Autodesk Inventor part; units mm, degrees
(part 2 of 2)
  measures "d144" distance between parallel lines of L36 L56
  measures "d146" radius of A87
  measures "d147" diameter of A91
  measures "d148" distance between parallel lines of L36 L60
  measures "d149" distance between parallel lines of L22 L61
  measures "d150" distance between parallel lines of L31 L62
  measures "d151" radius of A94
  measures "d153" distance between parallel lines of L21 L63
  measures "d154" distance between parallel lines of L22 L64
  measures "d155" distance between parallel lines of L38 L65
  measures "d156" distance between parallel lines of L23 L66
  measures "d157" radius of A101
  measures "d158" radius of A107
  measures "d159" diameter of A108
  measures "d160" distance between parallel lines of L32 L68
  measures "d161" distance between parallel lines of L28 L69
  measures "d162" distance between parallel lines of L29 L70
  measures "d163" distance between parallel lines of L30 L71
  measures "d164" radius of A112
  measures "d170" distance between parallel lines of L26 L73
  measures "d171" distance between parallel lines of L29 L74
  measures "d172" radius of A117
  measures "d173" radius of A120
  measures "d174" diameter of A122
  measures "d175" distance between parallel lines of L23 L76
  measures "d176" distance between parallel lines of L27 L77
  measures "d177" distance between parallel lines of L26 L78
  measures "d178" distance between parallel lines of L25 L79
extrude "Extrusion3" cut sketch "Sketch2" against normal blind 4.7625
sketch "Sketch4" plane through (0, 4.7625, 0) normal (0, 1, 0) x (1, 0, 0)
  arc A0 (-39.1165, 26.3357) -> (-36.1072, 19.7253) centre (-34.8076, 24.3071) ccw projected
  line L0 (-39.1165, 26.3357) -> (-33.046, 39.2298) projected
  arc A1 (-24.1207, 38.3715) -> (-33.046, 39.2298) centre (-28.7371, 37.2012) ccw projected
  line L1 (-24.1207, 38.3715) -> (-20.9678, 25.9338) projected
  arc A2 (-25.5116, 20.0016) -> (-20.9678, 25.9338) centre (-25.5843, 24.7636) ccw projected
  arc A3 (-25.5116, 20.0016) -> (-29.2434, 18.9092) centre (-25.4, 12.7) ccw projected
  arc A4 (-34.2566, 18.9092) -> (-29.2434, 18.9092) centre (-31.75, 22.9587) ccw projected
  arc A5 (-34.2566, 18.9092) -> (-36.1072, 19.7253) centre (-38.1, 12.7) ccw projected
  arc A6 (10.7493, 83.4364) -> (18.6675, 82.9982) centre (14.8541, 85.8512) ccw projected
  line L2 (10.7493, 83.4364) -> (3.5125, 95.7378) projected
  arc A7 (5.2361, 102.2771) -> (3.5125, 95.7378) centre (7.6174, 98.1526) ccw projected
  line L3 (5.2361, 102.2771) -> (9.4199, 104.6926) projected
  arc A8 (13.3535, 105.0706) -> (9.4199, 104.6926) centre (11.8012, 100.5682) ccw projected
  arc A9 (13.3535, 105.0706) -> (19.7173, 105.0706) centre (16.5354, 114.3) ccw projected
  arc A10 (23.6509, 104.6926) -> (19.7173, 105.0706) centre (21.2696, 100.5682) ccw projected
  line L4 (23.6509, 104.6926) -> (26.8599, 102.8399) projected
  arc A11 (28.292, 95.8625) -> (26.8599, 102.8399) centre (24.4786, 98.7155) ccw projected
  line L5 (28.292, 95.8625) -> (18.6675, 82.9982) projected
  arc A12 (33.2042, 118.4244) -> (33.2042, 110.1756) centre (35.5854, 114.3) ccw projected
  line L6 (33.2042, 118.4244) -> (34.5005, 119.1729) projected
  arc A13 (37.5333, 119.7662) -> (34.5005, 119.1729) centre (36.8818, 115.0485) ccw projected
  arc A14 (37.5333, 119.7662) -> (40.1924, 119.8887) centre (38.5324, 127) ccw projected
  arc A15 (46.0375, 115.2508) -> (40.1924, 119.8887) centre (41.275, 115.2508) ccw projected
  line L7 (46.0375, 115.2508) -> (46.0375, 114.3) projected
  arc A16 (39.6449, 108.8173) -> (46.0375, 114.3) centre (40.49, 114.3) ccw projected
  arc A17 (39.6449, 108.8173) -> (37.5333, 108.8338) centre (38.5324, 101.6) ccw projected
  arc A18 (34.5005, 109.4271) -> (37.5333, 108.8338) centre (36.8818, 113.5515) ccw projected
  line L8 (34.5005, 109.4271) -> (33.2042, 110.1756) projected
  arc A19 (-0.6991, 113.9403) -> (2.8442, 111.8946) centre (1.6631, 113.9403) ccw projected
  line L9 (-0.6991, 113.9403) -> (-0.6991, 114.6597) projected
  arc A20 (2.8442, 116.7054) -> (-0.6991, 114.6597) centre (1.6631, 114.6597) ccw projected
  line L10 (2.8442, 116.7054) -> (3.4671, 116.3457) projected
  arc A21 (3.4671, 112.2543) -> (3.4671, 116.3457) centre (2.286, 114.3) ccw projected
  line L11 (3.4671, 112.2543) -> (2.8442, 111.8946) projected
  line L12 (41.275, 207.9625) -> (30.1653, 207.9625) projected
  arc A22 (26.0308, 215.0888) -> (30.1653, 207.9625) centre (30.1653, 212.725) ccw projected
  line L13 (26.0308, 215.0888) -> (37.1405, 234.5209) projected
  arc A23 (46.0375, 232.1571) -> (37.1405, 234.5209) centre (41.275, 232.1571) ccw projected
  line L14 (46.0375, 232.1571) -> (46.0375, 212.725) projected
  arc A24 (41.275, 207.9625) -> (46.0375, 212.725) centre (41.275, 212.725) ccw projected
  line L15 (-18.8398, 318.7446) -> (-15.9012, 313.5602) projected
  arc A25 (-18.9742, 306.5711) -> (-15.9012, 313.5602) centre (-20.0445, 311.2118) ccw projected
  line L16 (-18.9742, 306.5711) -> (-23.6444, 305.494) projected
  arc A26 (-29.3048, 311.4041) -> (-23.6444, 305.494) centre (-24.7146, 310.1347) ccw projected
  line L17 (-29.3048, 311.4041) -> (-27.5732, 317.6656) projected
  arc A27 (-18.8398, 318.7446) -> (-27.5732, 317.6656) centre (-22.983, 316.3962) ccw projected
  arc A28 (-53.975, 336.3341) -> (-58.7375, 331.5716) centre (-53.975, 331.5716) ccw projected
  line L18 (-53.975, 336.3341) -> (-47.8591, 336.3341) projected
  arc A29 (-43.4942, 333.4766) -> (-47.8591, 336.3341) centre (-47.8591, 331.5716) ccw projected
  arc A30 (-43.4942, 333.4766) -> (-38.0327, 326.2997) centre (-26.0346, 341.0966) ccw projected
  arc A31 (-36.442, 321.3311) -> (-38.0327, 326.2997) centre (-41.0322, 322.6005) ccw projected
  line L19 (-36.442, 321.3311) -> (-40.7412, 305.7855) projected
  arc A32 (-43.8878, 302.5165) -> (-40.7412, 305.7855) centre (-45.3314, 307.055) ccw projected
  line L20 (-43.8878, 302.5165) -> (-52.3056, 299.8389) projected
  arc A33 (-52.3056, 299.8389) -> (-52.4379, 299.7953) centre (-50.2604, 293.4095) ccw projected
  arc A34 (-58.7375, 304.3029) -> (-52.4379, 299.7953) centre (-53.975, 304.3029) ccw projected
  line L21 (-58.7375, 304.3029) -> (-58.7375, 331.5716) projected
  arc A35 (5.8207, 343.1819) -> (9.0856, 344.1221) centre (6.222, 347.9275) ccw projected
  line L22 (5.8207, 343.1819) -> (-3.8863, 344.0029) projected
  arc A36 (-7.9949, 347.2181) -> (-3.8863, 344.0029) centre (-3.485, 348.7485) ccw projected
  arc A37 (-7.9949, 347.2181) -> (-14.358, 356.1485) centre (-26.0346, 341.0966) ccw projected
  arc A38 (-16.0554, 361.0817) -> (-14.358, 356.1485) centre (-11.4389, 359.9115) ccw projected
  line L23 (-16.0554, 361.0817) -> (-13.3658, 371.6918) projected
  arc A39 (-4.8645, 373.2765) -> (-13.3658, 371.6918) centre (-8.7493, 370.5216) ccw projected
  line L24 (-4.8645, 373.2765) -> (10.8092, 351.1749) projected
  arc A40 (9.5261, 344.431) -> (10.8092, 351.1749) centre (6.9244, 348.42) ccw projected
  arc A41 (9.5261, 344.431) -> (9.0856, 344.1221) centre (13.904, 337.7188) ccw projected
  arc A42 (-9.4515, 321.4974) -> (-1.2033, 321.431) centre (-5.3082, 323.8458) ccw projected
  line L25 (-9.4515, 321.4974) -> (-11.1297, 324.4583) projected
  arc A43 (-10.796, 329.6646) -> (-11.1297, 324.4583) centre (-6.9864, 326.8067) ccw projected
  arc A44 (-10.796, 329.6646) -> (-9.2793, 332.0323) centre (-26.0346, 341.0966) ccw projected
  arc A45 (-4.6891, 334.5118) -> (-9.2793, 332.0323) centre (-5.0904, 329.7662) ccw projected
  line L26 (-4.6891, 334.5118) -> (-1.5787, 334.2487) projected
  arc A46 (2.1248, 327.0883) -> (-1.5787, 334.2487) centre (-1.9801, 329.5032) ccw projected
  line L27 (2.1248, 327.0883) -> (-1.2033, 321.431) projected
  arc A47 (19.7173, 301.3294) -> (13.3535, 301.3294) centre (16.5354, 292.1) ccw projected
  arc A48 (9.4199, 301.7074) -> (13.3535, 301.3294) centre (11.8012, 305.8318) ccw projected
  line L28 (9.4199, 301.7074) -> (5.2361, 304.1229) projected
  arc A49 (3.5125, 310.6622) -> (5.2361, 304.1229) centre (7.6174, 308.2474) ccw projected
  line L29 (3.5125, 310.6622) -> (10.7493, 322.9636) projected
  arc A50 (18.6675, 323.4018) -> (10.7493, 322.9636) centre (14.8541, 320.5488) ccw projected
  line L30 (18.6675, 323.4018) -> (28.292, 310.5375) projected
  arc A51 (26.8599, 303.5601) -> (28.292, 310.5375) centre (24.4786, 307.6845) ccw projected
  line L31 (26.8599, 303.5601) -> (23.6509, 301.7074) projected
  arc A52 (19.7173, 301.3294) -> (23.6509, 301.7074) centre (21.2696, 305.8318) ccw projected
  arc A53 (9.6134, 220.0272) -> (17.8824, 220.0272) centre (13.7479, 222.3909) ccw projected
  line L32 (9.6134, 220.0272) -> (4.0277, 229.7971) projected
  arc A54 (4.342, 235.0047) -> (4.0277, 229.7971) centre (8.1622, 232.1609) ccw projected
  arc A55 (4.342, 235.0047) -> (7.636, 242.1522) centre (-10.9389, 246.38) ccw projected
  arc A56 (11.391, 245.774) -> (7.636, 242.1522) centre (12.2798, 241.0952) ccw projected
  line L33 (11.391, 245.774) -> (25.0344, 248.3657) projected
  arc A57 (30.0577, 241.3231) -> (25.0344, 248.3657) centre (25.9232, 243.6869) ccw projected
  line L34 (30.0577, 241.3231) -> (17.8824, 220.0272) projected
  arc A58 (30.1653, 198.4375) -> (26.0308, 191.3112) centre (30.1653, 193.675) ccw projected
  line L35 (30.1653, 198.4375) -> (41.275, 198.4375) projected
  arc A59 (46.0375, 193.675) -> (41.275, 198.4375) centre (41.275, 193.675) ccw projected
  line L36 (46.0375, 193.675) -> (46.0375, 174.2429) projected
  arc A60 (37.1405, 171.8791) -> (46.0375, 174.2429) centre (41.275, 174.2429) ccw projected
  line L37 (37.1405, 171.8791) -> (26.0308, 191.3112) projected
  arc A61 (-58.7375, 140.2762) -> (-54.2943, 135.5245) centre (-53.975, 140.2762) ccw projected
  line L38 (-58.7375, 140.2762) -> (-58.7375, 193.675) projected
  arc A62 (-53.975, 198.4375) -> (-58.7375, 193.675) centre (-53.975, 193.675) ccw projected
  line L39 (-53.975, 198.4375) -> (-52.8865, 198.4375) projected
  arc A63 (-49.7125, 197.2256) -> (-52.8865, 198.4375) centre (-52.8865, 193.675) ccw projected
  arc A64 (-49.7125, 197.2256) -> (-45.8257, 195.3193) centre (-44.3715, 203.2) ccw projected
  arc A65 (-42.9243, 193.5516) -> (-45.8257, 195.3193) centre (-46.69, 190.6359) ccw projected
  line L40 (-42.9243, 193.5516) -> (-28.0657, 174.361) projected
  arc A66 (-27.6529, 169.1603) -> (-28.0657, 174.361) centre (-31.8314, 171.4453) ccw projected
  arc A67 (-27.6529, 169.1603) -> (-29.5057, 155.7567) centre (-10.9389, 160.02) ccw projected
  arc A68 (-31.3139, 150.863) -> (-29.5057, 155.7567) centre (-34.1474, 154.6908) ccw projected
  line L41 (-31.3139, 150.863) -> (-50.8212, 136.4228) projected
  arc A69 (-54.0935, 135.5084) -> (-50.8212, 136.4228) centre (-53.6548, 140.2507) ccw projected
  arc A70 (-54.0935, 135.5084) -> (-54.2943, 135.5245) centre (-54.8316, 127.5288) ccw projected
  arc A71 (-11.1297, 81.9417) -> (-10.796, 76.7354) centre (-6.9864, 79.5933) ccw projected
  line L42 (-11.1297, 81.9417) -> (-9.4515, 84.9026) projected
  arc A72 (-1.2033, 84.969) -> (-9.4515, 84.9026) centre (-5.3082, 82.5542) ccw projected
  line L43 (-1.2033, 84.969) -> (2.1248, 79.3117) projected
  arc A73 (-1.5787, 72.1513) -> (2.1248, 79.3117) centre (-1.9801, 76.8968) ccw projected
  line L44 (-1.5787, 72.1513) -> (-4.6891, 71.8882) projected
  arc A74 (-9.2793, 74.3677) -> (-4.6891, 71.8882) centre (-5.0904, 76.6338) ccw projected
  arc A75 (-9.2793, 74.3677) -> (-10.796, 76.7354) centre (-26.0346, 65.3034) ccw projected
  arc A76 (-53.975, 60.5409) -> (-58.7375, 55.7784) centre (-53.975, 55.7784) ccw projected
  line L45 (-53.975, 60.5409) -> (-47.8591, 60.5409) projected
  arc A77 (-43.4942, 57.6834) -> (-47.8591, 60.5409) centre (-47.8591, 55.7784) ccw projected
  arc A78 (-43.4942, 57.6834) -> (-40.3657, 52.7526) centre (-26.0346, 65.3034) ccw projected
  arc A79 (-39.6396, 47.5863) -> (-40.3657, 52.7526) centre (-43.9484, 49.6149) ccw projected
  line L46 (-39.6396, 47.5863) -> (-49.6661, 26.2893) projected
  arc A80 (-58.7375, 28.3179) -> (-49.6661, 26.2893) centre (-53.975, 28.3179) ccw projected
  line L47 (-58.7375, 28.3179) -> (-58.7375, 55.7784) projected
  arc A81 (-13.3658, 34.7082) -> (-4.8645, 33.1235) centre (-8.7493, 35.8784) ccw projected
  line L48 (-13.3658, 34.7082) -> (-16.0554, 45.3183) projected
  arc A82 (-14.358, 50.2515) -> (-16.0554, 45.3183) centre (-11.4389, 46.4885) ccw projected
  arc A83 (-14.358, 50.2515) -> (-7.9949, 59.1819) centre (-26.0346, 65.3034) ccw projected
  arc A84 (-3.8863, 62.3971) -> (-7.9949, 59.1819) centre (-3.485, 57.6515) ccw projected
  line L49 (-3.8863, 62.3971) -> (5.8207, 63.2181) projected
  arc A85 (9.0856, 62.2779) -> (5.8207, 63.2181) centre (6.222, 58.4725) ccw projected
  arc A86 (9.0856, 62.2779) -> (9.5261, 61.969) centre (13.904, 68.6812) ccw projected
  arc A87 (10.8092, 55.2251) -> (9.5261, 61.969) centre (6.9244, 57.98) ccw projected
  line L50 (10.8092, 55.2251) -> (-4.8645, 33.1235) projected
  arc A88 (-12.0658, 137.7103) -> (-15.5991, 141.5488) centre (-16.7641, 136.931) ccw projected
  line L51 (-12.0658, 137.7103) -> (-11.3718, 133.5261) projected
  arc A89 (-11.8825, 130.4783) -> (-11.3718, 133.5261) centre (-16.0701, 132.7468) ccw projected
  arc A90 (-11.8825, 130.4783) -> (-11.2268, 122.5178) centre (-5.4616, 127) ccw projected
  arc A91 (-10.2241, 119.5947) -> (-11.2268, 122.5178) centre (-14.9866, 119.5947) ccw projected
  line L52 (-10.2241, 119.5947) -> (-10.2241, 113.5718) projected
  arc A92 (-16.0569, 108.9311) -> (-10.2241, 113.5718) centre (-14.9866, 113.5718) ccw projected
  line L53 (-16.0569, 108.9311) -> (-30.7922, 112.3296) projected
  arc A93 (-33.2127, 113.7305) -> (-30.7922, 112.3296) centre (-29.7219, 116.9703) ccw projected
  arc A94 (-33.2127, 113.7305) -> (-36.1128, 115.5703) centre (-38.1579, 109.1408) ccw projected
  line L54 (-36.1128, 115.5703) -> (-44.4253, 118.2144) projected
  arc A95 (-47.3989, 124.5331) -> (-44.4253, 118.2144) centre (-42.9817, 122.7528) ccw projected
  arc A96 (-47.3989, 124.5331) -> (-46.9843, 125.9045) centre (-54.8316, 127.5288) ccw projected
  arc A97 (-45.1542, 128.7671) -> (-46.9843, 125.9045) centre (-42.3206, 124.9392) ccw projected
  line L55 (-45.1542, 128.7671) -> (-25.6468, 143.2073) projected
  arc A98 (-20.4384, 143.5075) -> (-25.6468, 143.2073) centre (-22.8133, 139.3794) ccw projected
  arc A99 (-20.4384, 143.5075) -> (-15.5991, 141.5488) centre (-10.9389, 160.02) ccw projected
  arc A100 (-20.5343, 180.1922) -> (-15.6027, 178.4903) centre (-16.7686, 183.1079) ccw projected
  line L56 (-20.5343, 180.1922) -> (-28.716, 190.7594) projected
  arc A101 (-24.9504, 198.4375) -> (-28.716, 190.7594) centre (-24.9504, 193.675) ccw projected
  line L57 (-24.9504, 198.4375) -> (-2.6695, 198.4375) projected
  arc A102 (1.465, 191.3112) -> (-2.6695, 198.4375) centre (-2.6695, 193.675) ccw projected
  line L58 (1.465, 191.3112) -> (-4.2413, 181.3304) projected
  arc A103 (-8.8884, 178.9593) -> (-4.2413, 181.3304) centre (-8.3758, 183.6942) ccw projected
  arc A104 (-8.8884, 178.9593) -> (-15.6027, 178.4903) centre (-10.9389, 160.02) ccw projected
  arc A105 (-52.8865, 207.9625) -> (-49.7125, 209.1744) centre (-52.8865, 212.725) ccw projected
  line L59 (-52.8865, 207.9625) -> (-53.975, 207.9625) projected
  arc A106 (-58.7375, 212.725) -> (-53.975, 207.9625) centre (-53.975, 212.725) ccw projected
  line L60 (-58.7375, 212.725) -> (-58.7375, 266.1238) projected
  arc A107 (-54.2943, 270.8755) -> (-58.7375, 266.1238) centre (-53.975, 266.1238) ccw projected
  arc A108 (-54.2943, 270.8755) -> (-54.0935, 270.8916) centre (-54.8316, 278.8712) ccw projected
  arc A109 (-50.8212, 269.9772) -> (-54.0935, 270.8916) centre (-53.6548, 266.1493) ccw projected
  line L61 (-50.8212, 269.9772) -> (-31.3139, 255.537) projected
  arc A110 (-29.5057, 250.6433) -> (-31.3139, 255.537) centre (-34.1474, 251.7092) ccw projected
  arc A111 (-29.5057, 250.6433) -> (-27.6529, 237.2397) centre (-10.9389, 246.38) ccw projected
  arc A112 (-28.0657, 232.039) -> (-27.6529, 237.2397) centre (-31.8314, 234.9547) ccw projected
  line L62 (-28.0657, 232.039) -> (-42.9243, 212.8484) projected
  arc A113 (-45.8257, 211.0807) -> (-42.9243, 212.8484) centre (-46.69, 215.7641) ccw projected
  arc A114 (-45.8257, 211.0807) -> (-49.7125, 209.1744) centre (-44.3715, 203.2) ccw projected
  arc A115 (33.5298, 259.6748) -> (37.2468, 265.565) centre (32.641, 264.3536) ccw projected
  line L63 (33.5298, 259.6748) -> (9.6134, 255.1317) projected
  arc A116 (4.792, 257.1244) -> (9.6134, 255.1317) centre (8.7247, 259.8105) ccw projected
  arc A117 (4.792, 257.1244) -> (-0.5645, 262.3573) centre (-10.9389, 246.38) ccw projected
  arc A118 (-2.6692, 267.131) -> (-0.5645, 262.3573) centre (2.0291, 266.3516) ccw projected
  line L64 (-2.6692, 267.131) -> (-1.9752, 271.3152) projected
  arc A119 (-0.5077, 274.0348) -> (-1.9752, 271.3152) centre (2.7231, 270.5358) ccw projected
  arc A120 (-0.5077, 274.0348) -> (1.3026, 276.6483) centre (-5.4616, 279.4) ccw projected
  arc A121 (3.3328, 278.9782) -> (1.3026, 276.6483) centre (5.714, 274.8538) ccw projected
  line L65 (3.3328, 278.9782) -> (9.4199, 282.4926) projected
  arc A122 (13.3535, 282.8706) -> (9.4199, 282.4926) centre (11.8012, 278.3682) ccw projected
  arc A123 (13.3535, 282.8706) -> (19.7173, 282.8706) centre (16.5354, 292.1) ccw projected
  arc A124 (23.6509, 282.4926) -> (19.7173, 282.8706) centre (21.2696, 278.3682) ccw projected
  line L66 (23.6509, 282.4926) -> (29.738, 278.9782) projected
  arc A125 (31.7682, 276.6483) -> (29.738, 278.9782) centre (27.3568, 274.8538) ccw projected
  arc A126 (31.7682, 276.6483) -> (34.0971, 273.5988) centre (38.5324, 279.4) ccw projected
  arc A127 (35.8103, 271.0268) -> (34.0971, 273.5988) centre (31.2044, 269.8154) ccw projected
  line L67 (35.8103, 271.0268) -> (37.2468, 265.565) projected
  line L68 (2.8442, 294.5054) -> (3.4671, 294.1457) projected
  arc A128 (3.4671, 290.0543) -> (3.4671, 294.1457) centre (2.286, 292.1) ccw projected
  line L69 (3.4671, 290.0543) -> (2.8442, 289.6946) projected
  arc A129 (-0.6991, 291.7403) -> (2.8442, 289.6946) centre (1.6631, 291.7403) ccw projected
  line L70 (-0.6991, 291.7403) -> (-0.6991, 292.4597) projected
  arc A130 (2.8442, 294.5054) -> (-0.6991, 292.4597) centre (1.6631, 292.4597) ccw projected
  arc A131 (-29.2434, 387.4908) -> (-25.5116, 386.3984) centre (-25.4, 393.7) ccw projected
  arc A132 (-20.9678, 380.4662) -> (-25.5116, 386.3984) centre (-25.5843, 381.6364) ccw projected
  line L71 (-20.9678, 380.4662) -> (-24.1207, 368.0285) projected
  arc A133 (-33.046, 367.1702) -> (-24.1207, 368.0285) centre (-28.7371, 369.1988) ccw projected
  line L72 (-33.046, 367.1702) -> (-39.1165, 380.0643) projected
  arc A134 (-36.1072, 386.6747) -> (-39.1165, 380.0643) centre (-34.8076, 382.0929) ccw projected
  arc A135 (-36.1072, 386.6747) -> (-34.2566, 387.4908) centre (-38.1, 393.7) ccw projected
  arc A136 (-29.2434, 387.4908) -> (-34.2566, 387.4908) centre (-31.75, 383.4413) ccw projected
  arc A137 (-49.6661, 380.1107) -> (-58.7375, 378.0821) centre (-53.975, 378.0821) ccw projected
  line L73 (-49.6661, 380.1107) -> (-39.6396, 358.8137) projected
  arc A138 (-40.3657, 353.6474) -> (-39.6396, 358.8137) centre (-43.9484, 356.7851) ccw projected
  arc A139 (-40.3657, 353.6474) -> (-43.4942, 348.7166) centre (-26.0346, 341.0966) ccw projected
  arc A140 (-47.8591, 345.8591) -> (-43.4942, 348.7166) centre (-47.8591, 350.6216) ccw projected
  line L74 (-47.8591, 345.8591) -> (-53.975, 345.8591) projected
  arc A141 (-58.7375, 350.6216) -> (-53.975, 345.8591) centre (-53.975, 350.6216) ccw projected
  line L75 (-58.7375, 350.6216) -> (-58.7375, 378.0821) projected
  arc A142 (34.5005, 287.2271) -> (37.5333, 286.6338) centre (36.8818, 291.3515) ccw projected
  line L76 (34.5005, 287.2271) -> (33.2042, 287.9756) projected
  arc A143 (33.2042, 296.2244) -> (33.2042, 287.9756) centre (35.5854, 292.1) ccw projected
  line L77 (33.2042, 296.2244) -> (34.5005, 296.9729) projected
  arc A144 (37.5333, 297.5662) -> (34.5005, 296.9729) centre (36.8818, 292.8485) ccw projected
  arc A145 (37.5333, 297.5662) -> (39.6449, 297.5827) centre (38.5324, 304.8) ccw projected
  arc A146 (46.0375, 292.1) -> (39.6449, 297.5827) centre (40.49, 292.1) ccw projected
  line L78 (46.0375, 292.1) -> (46.0375, 291.1492) projected
  arc A147 (40.1924, 286.5113) -> (46.0375, 291.1492) centre (41.275, 291.1492) ccw projected
  arc A148 (40.1924, 286.5113) -> (37.5333, 286.6338) centre (38.5324, 279.4) ccw projected
  arc A149 (-11.3718, 272.8739) -> (-11.8825, 275.9217) centre (-16.0701, 273.6532) ccw projected
  line L79 (-11.3718, 272.8739) -> (-12.0658, 268.6897) projected
  arc A150 (-15.5991, 264.8512) -> (-12.0658, 268.6897) centre (-16.7641, 269.469) ccw projected
  arc A151 (-15.5991, 264.8512) -> (-20.4384, 262.8925) centre (-10.9389, 246.38) ccw projected
  arc A152 (-25.6468, 263.1927) -> (-20.4384, 262.8925) centre (-22.8133, 267.0206) ccw projected
  line L80 (-25.6468, 263.1927) -> (-45.1542, 277.6329) projected
  arc A153 (-46.9843, 280.4955) -> (-45.1542, 277.6329) centre (-42.3206, 281.4608) ccw projected
  arc A154 (-46.9843, 280.4955) -> (-47.3989, 281.8669) centre (-54.8316, 278.8712) ccw projected
  arc A155 (-44.4253, 288.1856) -> (-47.3989, 281.8669) centre (-42.9817, 283.6472) ccw projected
  line L81 (-44.4253, 288.1856) -> (-36.1128, 290.8297) projected
  arc A156 (-36.1128, 290.8297) -> (-33.2127, 292.6695) centre (-38.1579, 297.2592) ccw projected
  arc A157 (-30.7922, 294.0704) -> (-33.2127, 292.6695) centre (-29.7219, 289.4297) ccw projected
  line L82 (-30.7922, 294.0704) -> (-16.0569, 297.4689) projected
  arc A158 (-10.2241, 292.8282) -> (-16.0569, 297.4689) centre (-14.9866, 292.8282) ccw projected
  line L83 (-10.2241, 292.8282) -> (-10.2241, 286.8053) projected
  arc A159 (-11.2268, 283.8822) -> (-10.2241, 286.8053) centre (-14.9866, 286.8053) ccw projected
  arc A160 (-11.2268, 283.8822) -> (-11.8825, 275.9217) centre (-5.4616, 279.4) ccw projected
  line L84 (-4.2413, 225.0696) -> (1.465, 215.0888) projected
  arc A161 (-2.6695, 207.9625) -> (1.465, 215.0888) centre (-2.6695, 212.725) ccw projected
  line L85 (-2.6695, 207.9625) -> (-24.9504, 207.9625) projected
  arc A162 (-28.716, 215.6406) -> (-24.9504, 207.9625) centre (-24.9504, 212.725) ccw projected
  line L86 (-28.716, 215.6406) -> (-20.5343, 226.2078) projected
  arc A163 (-15.6027, 227.9097) -> (-20.5343, 226.2078) centre (-16.7686, 223.2921) ccw projected
  arc A164 (-15.6027, 227.9097) -> (-8.8884, 227.4407) centre (-10.9389, 246.38) ccw projected
  arc A165 (-4.2413, 225.0696) -> (-8.8884, 227.4407) centre (-8.3758, 222.7058) ccw projected
  arc A166 (25.0344, 158.0343) -> (30.0577, 165.0769) centre (25.9232, 162.7131) ccw projected
  line L87 (25.0344, 158.0343) -> (11.391, 160.626) projected
  arc A167 (7.636, 164.2478) -> (11.391, 160.626) centre (12.2798, 165.3048) ccw projected
  arc A168 (7.636, 164.2478) -> (4.342, 171.3953) centre (-10.9389, 160.02) ccw projected
  arc A169 (4.0277, 176.6029) -> (4.342, 171.3953) centre (8.1622, 174.2391) ccw projected
  line L88 (4.0277, 176.6029) -> (9.6134, 186.3728) projected
  arc A170 (17.8824, 186.3728) -> (9.6134, 186.3728) centre (13.7479, 184.0091) ccw projected
  line L89 (17.8824, 186.3728) -> (30.0577, 165.0769) projected
  arc A171 (-1.9752, 135.0848) -> (-0.5077, 132.3652) centre (2.7231, 135.8642) ccw projected
  line L90 (-1.9752, 135.0848) -> (-2.6692, 139.269) projected
  arc A172 (-0.5645, 144.0427) -> (-2.6692, 139.269) centre (2.0291, 140.0484) ccw projected
  arc A173 (-0.5645, 144.0427) -> (4.792, 149.2756) centre (-10.9389, 160.02) ccw projected
  arc A174 (9.6134, 151.2683) -> (4.792, 149.2756) centre (8.7247, 146.5895) ccw projected
  line L91 (9.6134, 151.2683) -> (33.5298, 146.7252) projected
  arc A175 (37.2468, 140.835) -> (33.5298, 146.7252) centre (32.641, 142.0464) ccw projected
  line L92 (37.2468, 140.835) -> (35.8103, 135.3732) projected
  arc A176 (34.0971, 132.8012) -> (35.8103, 135.3732) centre (31.2044, 136.5846) ccw projected
  arc A177 (34.0971, 132.8012) -> (31.7682, 129.7517) centre (38.5324, 127) ccw projected
  arc A178 (29.738, 127.4218) -> (31.7682, 129.7517) centre (27.3568, 131.5462) ccw projected
  line L93 (29.738, 127.4218) -> (23.6509, 123.9074) projected
  arc A179 (19.7173, 123.5294) -> (23.6509, 123.9074) centre (21.2696, 128.0318) ccw projected
  arc A180 (19.7173, 123.5294) -> (13.3535, 123.5294) centre (16.5354, 114.3) ccw projected
  arc A181 (9.4199, 123.9074) -> (13.3535, 123.5294) centre (11.8012, 128.0318) ccw projected
  line L94 (9.4199, 123.9074) -> (3.3328, 127.4218) projected
  arc A182 (1.3026, 129.7517) -> (3.3328, 127.4218) centre (5.714, 131.5462) ccw projected
  arc A183 (1.3026, 129.7517) -> (-0.5077, 132.3652) centre (-5.4616, 127) ccw projected
  line L95 (-15.9012, 92.8398) -> (-18.8398, 87.6554) projected
  arc A184 (-27.5732, 88.7344) -> (-18.8398, 87.6554) centre (-22.983, 90.0038) ccw projected
  line L96 (-27.5732, 88.7344) -> (-29.3048, 94.9959) projected
  arc A185 (-23.6444, 100.906) -> (-29.3048, 94.9959) centre (-24.7146, 96.2653) ccw projected
  line L97 (-23.6444, 100.906) -> (-18.9742, 99.8289) projected
  arc A186 (-15.9012, 92.8398) -> (-18.9742, 99.8289) centre (-20.0445, 95.1882) ccw projected
  line L98 (-47.8591, 70.0659) -> (-53.975, 70.0659) projected
  arc A187 (-58.7375, 74.8284) -> (-53.975, 70.0659) centre (-53.975, 74.8284) ccw projected
  line L99 (-58.7375, 74.8284) -> (-58.7375, 102.0971) projected
  arc A188 (-52.4379, 106.6047) -> (-58.7375, 102.0971) centre (-53.975, 102.0971) ccw projected
  arc A189 (-52.4379, 106.6047) -> (-52.3056, 106.5611) centre (-50.2604, 112.9905) ccw projected
  line L100 (-52.3056, 106.5611) -> (-43.8878, 103.8835) projected
  arc A190 (-40.7412, 100.6145) -> (-43.8878, 103.8835) centre (-45.3314, 99.345) ccw projected
  line L101 (-40.7412, 100.6145) -> (-36.442, 85.0689) projected
  arc A191 (-38.0327, 80.1003) -> (-36.442, 85.0689) centre (-41.0322, 83.7995) ccw projected
  arc A192 (-38.0327, 80.1003) -> (-43.4942, 72.9234) centre (-26.0346, 65.3034) ccw projected
  arc A193 (-47.8591, 70.0659) -> (-43.4942, 72.9234) centre (-47.8591, 74.8284) ccw projected
  line L102 (-63.5, 401.6375) -> (-63.5, 4.7625) projected
  arc A194 (-63.5, 4.7625) -> (-58.7375, 0) centre (-58.7375, 4.7625) ccw projected
  line L103 (-58.7375, 0) -> (-4.7625, 0) projected
  arc A195 (-4.7625, 0) -> (0, 4.7625) centre (-4.7625, 4.7625) ccw projected
  line L104 (0, 4.7625) -> (0, 30.2327) projected
  arc A196 (0.8777, 32.9877) -> (0, 30.2327) centre (4.7625, 30.2327) ccw projected
  line L105 (0.8777, 32.9877) -> (44.4852, 94.479) projected
  arc A197 (44.4852, 94.479) -> (50.8, 114.3) centre (16.5354, 114.3) ccw projected
  line L106 (50.8, 114.3) -> (50.8, 292.1) projected
  arc A198 (50.8, 292.1) -> (44.4852, 311.921) centre (16.5354, 292.1) ccw projected
  line L107 (44.4852, 311.921) -> (0.8777, 373.4123) projected
  arc A199 (0, 376.1673) -> (0.8777, 373.4123) centre (4.7625, 376.1673) ccw projected
  line L108 (0, 376.1673) -> (0, 401.6375) projected
  arc A200 (0, 401.6375) -> (-4.7625, 406.4) centre (-4.7625, 401.6375) ccw projected
  line L109 (-4.7625, 406.4) -> (-58.7375, 406.4) projected
  arc A201 (-58.7375, 406.4) -> (-63.5, 401.6375) centre (-58.7375, 401.6375) ccw projected
  circle A202 centre (38.5324, 304.8) radius 2.54 projected
  circle A203 centre (-5.4616, 304.8) radius 2.54 projected
  circle A204 centre (-5.4616, 127) radius 2.54 projected
  circle A205 centre (38.5324, 127) radius 2.54 projected
  circle A206 centre (44.45, 256.9015) radius 3.2512 projected
  circle A207 centre (-44.3715, 203.2) radius 3.2512 projected
  circle A208 centre (44.45, 149.4985) radius 3.2512 projected
  circle A209 centre (-25.4, 393.7) radius 2.54 projected
  circle A210 centre (-50.8, 393.7) radius 2.54 projected
  circle A211 centre (-38.1, 12.7) radius 2.54 projected
  circle A212 centre (-26.0346, 65.3034) radius 14.2875 projected
  circle A213 centre (-26.0346, 341.0966) radius 14.2875 projected
  circle A214 centre (16.5354, 292.1) radius 5 projected
  circle A215 centre (16.5354, 114.3) radius 5 projected
  circle A216 centre (-10.9389, 160.02) radius 14.2875 projected
  circle A217 centre (-10.9389, 246.38) radius 14.2875 projected
  circle A218 centre (-12.7, 12.7) radius 2.54 projected
  circle A219 centre (-25.4, 12.7) radius 2.54 projected
  circle A220 centre (-50.8, 12.7) radius 2.54 projected
  circle A221 centre (-38.1, 393.7) radius 2.54 projected
  circle A222 centre (-12.7, 393.7) radius 2.54 projected
  circle A223 centre (-54.8316, 127.5288) radius 3.2512 projected
  circle A224 centre (-54.8316, 278.8712) radius 3.2512 projected
  circle A225 centre (38.5324, 101.6) radius 2.54 projected
  circle A226 centre (-5.4616, 101.6) radius 2.54 projected
  circle A227 centre (-5.4616, 279.4) radius 2.54 projected
  circle A228 centre (38.5324, 279.4) radius 2.54 projected
  circle A229 centre (13.904, 337.7188) radius 3.2512 projected
  circle A230 centre (13.904, 68.6812) radius 3.2512 projected
  line L110 (-50.8619, 295.3005) -> (-38.7594, 299.1502) projected
  arc A231 (-37.5564, 295.3682) -> (-38.7594, 299.1502) centre (-38.1579, 297.2592) ccw projected
  line L111 (-37.5564, 295.3682) -> (-49.6589, 291.5185) projected
  arc A232 (-50.8619, 295.3005) -> (-49.6589, 291.5185) centre (-50.2604, 293.4095) ccw projected
  line L112 (-49.6589, 114.8815) -> (-37.5564, 111.0318) projected
  arc A233 (-38.7594, 107.2498) -> (-37.5564, 111.0318) centre (-38.1579, 109.1408) ccw projected
  line L113 (-38.7594, 107.2498) -> (-50.8619, 111.0995) projected
  arc A234 (-49.6589, 114.8815) -> (-50.8619, 111.0995) centre (-50.2604, 112.9905) ccw projected
  line L114 (-19.2643, 40.8223) -> (-32.8049, 89.7845) construction
  circle A235 centre (-32.8049, 89.7845) radius 2.54
  circle A236 centre (-19.2643, 40.8223) radius 2.54
  line L115 (-44.3715, 203.2) -> (50.8, 203.2) construction
  circle A237 centre (-32.8049, 316.6155) radius 2.54
  circle A238 centre (-19.2643, 365.5777) radius 2.54
  point P0 (0, 0)
  dimension "d219" = 50.8
  dimension "d224" = 5.08
  constraints: 4 centre point, 4 end point, 3 coincident, 2 midpoint, 2 symmetric about line, 1 equal radius, 1 parallel, 2 other
  measures "d219" distance of L114.start L114.end
  measures "d224" diameter of A236
extrude "Extrusion4" cut sketch "Sketch4" against normal blind 25.4 contours A235 | A236 | A237 | A238
body "Solid1"
